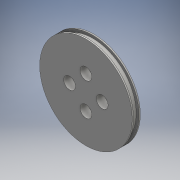
# Autodesk Inventor part: wheel
Saved by Autodesk Inventor 2016 (Build 200138000, 138)
## iProperties
Created: 2016-05-01
Part Number: wheel
Material: Generic
Document SubType Name: Modeling
Designer: mkepler
Density: 1 g/cm^3
Appearance: Default
Author: mkepler
Autodesk Inventor part; units mm, degrees
ref_plane "YZ Plane" through (0, 0, 0) normal (1, 0, 0) x (0, 1, 0)
ref_plane "XZ Plane" through (0, 0, 0) normal (0, 1, 0) x (-1, 0, 0)
ref_plane "XY Plane" through (0, 0, 0) normal (0, 0, 1) x (1, 0, 0)
sketch "Sketch1" plane through (0, 0, 0) normal (0, 1, 0) x (-1, 0, 0)
  circle A0 centre (0, 0) radius 17
  dimension "d0" = 34
  constraints: 1 centre point, 1 coincident
  measures "d0" diameter of A0
extrude "Extrusion1" add sketch "Sketch1" along normal blind 0.5
sketch "Sketch2" plane through (0, 0.5, 0) normal (0, 1, 0) x (1, 0, 0)
  circle A0 centre (0, 0) radius 16
  dimension "d3" = 32
  constraints: 1 centre point, 1 coincident
  measures "d3" diameter of A0
extrude "Extrusion2" add sketch "Sketch2" along normal blind 2
sketch "Sketch3" plane through (0, 2.5, 0) normal (0, 1, 0) x (1, 0, 0)
  circle A0 centre (0, 0) radius 17
  constraints: 1 centre point, 1 coincident
extrude "Extrusion3" add sketch "Sketch3" along normal blind 0.5
sketch "Sketch4" plane through (0, 3, 0) normal (0, 1, 0) x (1, 0, 0)
  circle A0 centre (0, -6) radius 2.175
  circle A1 centre (0, 6) radius 2.175
  circle A2 centre (6, 0) radius 2.175
  circle A3 centre (-6, 0) radius 2.175
  point P0 (0, 0)
  dimension "d8" = 4.35
  dimension "d9" = 6
  dimension "d10" = 4.35
  dimension "d11" = 6
  dimension "d12" = 4.35
  dimension "d13" = 6
  dimension "d14" = 4.35
  dimension "d15" = 6
  constraints: 4 centre point
  measures "d8" diameter of A0
  measures "d9" distance of point (0, 0) A0.centre
  measures "d10" diameter of A1
  measures "d11" distance of point (0, 0) A1.centre
  measures "d12" diameter of A2
  measures "d13" distance of point (0, 0) A2.centre
  measures "d14" diameter of A3
  measures "d15" distance of point (0, 0) A3.centre
hole "Hole1" at (6, 3, 0) at (0, 3, 6) at (-6, 3, 0) at (0, 3, -6) direction (0, -1, 0) diameter 4.35 end through all
body "Solid1"
